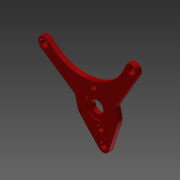
# Autodesk Inventor part: Part2
Saved by Autodesk Inventor 2014 SP1 (Build 180222100, 222)
## iProperties
Created: 2014-01-05
Part Number: Part2
Material: Aluminum 6061
Document SubType Name: Modeling
Designer: Rauhul Varma
Density: 2.71 g/cm^3
Appearance: Red
Mass: 9.68241 g
Surface Area: 32.817 cm^2
Volume: 3.57285 cm^3
Author: Rauhul Varma
Autodesk Inventor part; units mm, degrees
ref_plane "YZ Plane" through (0, 0, 0) normal (1, 0, 0) x (0, 1, 0)
ref_plane "XZ Plane" through (0, 0, 0) normal (0, 1, 0) x (-1, 0, 0)
ref_plane "XY Plane" through (0, 0, 0) normal (0, 0, 1) x (1, 0, 0)
sketch "Main Outline" plane through (0, 0, 0) normal (0, 0, 1) x (1, 0, 0)
  line L0 (0, 0) -> (304.8, 0) construction
  line L1 (304.8, 0) -> (304.8, 50.8) construction
  line L2 (304.8, 50.8) -> (0, 50.8) construction
  line L3 (0, 50.8) -> (0, 0) construction
  line L4 (0, 50.8) -> (0, 53.34) construction
  line L5 (0, 53.34) -> (304.8, 53.34) construction
  line L6 (304.8, 53.34) -> (304.8, 50.8) construction
  circle A0 centre (152.4, 23.8125) radius 17.4625 construction
  line L7 (152.4, 23.8125) -> (152.4, 0) construction
  circle A1 centre (152.4, 23.8125) radius 27.94 construction
  circle A2 centre (152.4, 23.8125) radius 21.59 construction
  line L8 (152.4, 23.8125) -> (144.1569, 60.2292) construction
  circle A3 centre (144.1569, 60.2292) radius 15.24 construction
  circle A4 centre (144.1569, 60.2292) radius 8.89 construction
  circle A5 centre (144.1569, 60.2292) radius 14.2875 construction
  arc A6 (163.8162, 72.0089) -> (128.198, 43.7805) centre (144.1569, 60.2292) ccw construction
  circle A7 centre (98.8106, 85.598) radius 32.258 construction
  circle A8 centre (124.5097, 147.0273) radius 32.258 construction
  circle A9 centre (174.158, 102.6533) radius 32.258 construction
  circle A10 centre (144.1569, 60.2292) radius 11.1125 construction
  circle A11 centre (152.4, 23.8125) radius 49.53 construction
  line L9 (144.1569, 60.2292) -> (124.5097, 147.0273) construction
  line L10 (144.1569, 60.2292) -> (98.8106, 85.598) construction
  line L11 (98.8106, 85.598) -> (174.158, 102.6533) construction
  line L12 (174.158, 102.6533) -> (144.1569, 60.2292) construction
  circle A12 centre (98.8106, 85.598) radius 9.5493 construction
  arc A13 (172.0498, 111.9669) -> (183.1109, 99.3313) centre (174.158, 102.6533) ccw construction
  circle A14 centre (124.5097, 147.0273) radius 9.5493 construction
  line L13 (96.7024, 94.9117) -> (172.0498, 111.9669) construction
  line L14 (183.1109, 99.3313) -> (165.6438, 52.2565) construction
  line L15 (92.161, 78.7444) -> (128.198, 43.7805) construction
  line L16 (172.0498, 111.9669) -> (174.158, 102.6533) construction
  line L17 (174.158, 102.6533) -> (183.1109, 99.3313) construction
  arc A15 (183.1109, 99.3313) -> (172.0498, 111.9669) centre (174.158, 102.6533) ccw construction
  arc A16 (165.6438, 52.2565) -> (163.8162, 72.0089) centre (144.1569, 60.2292) ccw construction
  arc A17 (128.198, 43.7805) -> (165.6438, 52.2565) centre (144.1569, 60.2292) ccw construction
  circle A18 centre (124.4396, 147.337) radius 32.258 construction
  circle A19 centre (124.3695, 147.6466) radius 32.258 construction
  circle A20 centre (124.2994, 147.9563) radius 32.258 construction
  line L18 (124.5097, 147.0273) -> (124.2994, 147.9563) construction
  circle A21 centre (124.5798, 146.7176) radius 32.258 construction
  circle A22 centre (117.4622, 43.2997) radius 9.525 construction
  circle A23 centre (175.54, 56.4459) radius 9.525 construction
  line L19 (152.4, 23.8125) -> (117.4622, 43.2997) construction
  line L20 (152.4, 23.8125) -> (175.54, 56.4459) construction
  line L21 (117.4622, 43.2997) -> (98.8106, 85.598) construction
  line L22 (175.54, 56.4459) -> (174.158, 102.6533) construction
  circle A24 centre (133.7342, 106.2753) radius 7.9375 construction
  line L23 (133.401, 150.5107) -> (165.496, 68.5894) construction
  circle A25 centre (152.4, 23.8125) radius 29.845 construction
  line L24 (114.985, 146.3422) -> (121.2977, 58.5849) construction
  circle A26 centre (99.0876, 85.443) radius 32.258 construction
  circle A27 centre (97.9793, 86.063) radius 32.258 construction
  line L25 (97.9793, 86.063) -> (98.8106, 85.598) construction
  circle A28 centre (98.2564, 85.908) radius 32.258 construction
  circle A29 centre (98.5335, 85.753) radius 32.258 construction
  circle A30 centre (152.4, 23.8125) radius 29.845 construction
  circle A31 centre (122.555, 23.8125) radius 6.35 construction
  circle A32 centre (179.3358, 36.6651) radius 6.35 construction
  line L26 (122.555, 23.8125) -> (152.4, 23.8125) construction
  line L27 (152.4, 23.8125) -> (182.245, 23.8125) construction
  circle A33 centre (182.245, 23.8125) radius 6.35 construction
  circle A34 centre (125.4642, 10.9599) radius 6.35 construction
  circle A35 centre (150.1885, 33.5827) radius 39.8623 construction
  line L28 (72.8944, 65.7819) -> (119.1902, 8.5205) construction
  circle A36 centre (174.708, 103.431) radius 32.258 construction
  line L29 (174.158, 102.6533) -> (174.708, 103.431) construction
  circle A37 centre (174.5246, 103.1717) radius 32.258 construction
  circle A38 centre (174.3413, 102.9125) radius 32.258 construction
  circle A39 centre (173.9747, 102.394) radius 32.258 construction
  line L30 (188.958, 24.3128) -> (206.0816, 95.9295) construction
  circle A40 centre (133.7342, 106.2753) radius 8.1693 construction
  arc A41 (85.4541, 115.7901) -> (94.2274, 135.7949) centre (79.2901, 130.4196) ccw construction
  arc A42 (156.6774, 149.9308) -> (173.2104, 135.6542) centre (172.4734, 151.5121) ccw construction
  line L31 (124.2994, 147.9563) -> (124.8602, 145.479) construction
  line L32 (114.3901, 145.7133) -> (114.9509, 143.236) construction
  line L33 (134.7695, 147.722) -> (134.2088, 150.1993) construction
  arc A43 (134.2088, 150.1993) -> (114.3901, 145.7133) centre (124.2994, 147.9563) ccw construction
  arc A44 (114.9509, 143.236) -> (134.7695, 147.722) centre (124.8602, 145.479) ccw construction
  line L34 (174.708, 103.431) -> (173.2414, 101.3571) construction
  line L35 (166.4126, 109.2972) -> (164.9461, 107.2234) construction
  line L36 (181.5368, 95.4909) -> (183.0033, 97.5647) construction
  arc A45 (183.0033, 97.5647) -> (166.4126, 109.2972) centre (174.708, 103.431) ccw construction
  arc A46 (164.9461, 107.2234) -> (181.5368, 95.4909) centre (173.2414, 101.3571) ccw construction
  line L37 (97.9793, 86.063) -> (100.196, 84.8229) construction
  line L38 (93.0188, 77.1963) -> (95.2355, 75.9562) construction
  line L39 (105.1564, 93.6897) -> (102.9398, 94.9298) construction
  arc A47 (102.9398, 94.9298) -> (93.0188, 77.1963) centre (97.9793, 86.063) ccw construction
  arc A48 (95.2355, 75.9562) -> (105.1564, 93.6897) centre (100.196, 84.8229) ccw construction
  circle A49 centre (117.4622, 43.2997) radius 3.9687 construction
  circle A50 centre (175.54, 56.4459) radius 3.9687 construction
  line L40 (152.4, 23.8125) -> (158.9889, -5.2961) construction
  arc A51 (89.3511, 54.6895) -> (85.9237, 49.6664) centre (88.3927, 51.6626) ccw construction
  arc A52 (201.2624, 75.7739) -> (196.006, 78.8314) centre (198.1744, 76.5122) ccw construction
  circle A53 centre (152.4, 23.8125) radius 14.224 construction
  circle A54 centre (133.7342, 106.2753) radius 3.9687 construction
  circle A55 centre (156.886, 3.9939) radius 6.35 construction
  circle A56 centre (156.886, 3.9939) radius 2.0828 construction
  circle A57 centre (152.4, 23.8125) radius 20.32 construction
  line L41 (132.9935, 29.8368) -> (152.4, 23.8125) construction
  line L42 (152.4, 23.8125) -> (167.3204, 37.6068) construction
  circle A58 centre (167.3204, 37.6068) radius 2.0828 construction
  circle A59 centre (167.3204, 37.6068) radius 3.9687 construction
  circle A60 centre (132.9935, 29.8368) radius 2.0828 construction
  circle A61 centre (132.9935, 29.8368) radius 3.9688 construction
  point P0 (173.9747, 102.394)
  point P1 (99.0876, 85.443)
  dimension "d18" = 99.06
  dimension "d58" = 64.516
  dimension "d86" = 64.516
  dimension "d0" = 304.8
  dimension "d1" = 50.8
  dimension "d2" = 2.54
  dimension "d3" = 34.925
  dimension "d4" = 23.8125
  dimension "d5" = 152.4
  dimension "d6" = 55.88
  dimension "d7" = 43.18
  dimension "d8" = 37.338
  dimension "d10" = 30.48
  dimension "d11" = 17.78
  dimension "d12" = 28.575
  dimension "d13" = 45.8366
  dimension "d14" = 64.516
  dimension "d15" = 64.516
  dimension "d16" = 64.516
  dimension "d17" = 22.225
  dimension "d19" = 51.9602
  dimension "d20" = 88.9939
  dimension "d21" = 19.0986
  dimension "d22" = 19.0986
  dimension "d23" = 19.0986
  dimension "d30" = 123.112
  dimension "d40" = 64.516
  dimension "d41" = 64.516
  dimension "d42" = 64.516
  dimension "d43" = 0.9525
  dimension "d44" = 0.3175
  dimension "d45" = 0.635
  dimension "d46" = 64.516
  dimension "d47" = 0.3175
  dimension "d48" = 19.05
  dimension "d49" = 19.05
  dimension "d50" = 40.005
  dimension "d51" = 40.005
  dimension "d52" = 46.228
  dimension "d54" = 46.228
  dimension "d55" = 15.875
  dimension "d56" = 41.4655
  dimension "d57" = 59.69
  dimension "d59" = 64.516
  dimension "d60" = 64.516
  dimension "d61" = 64.516
  dimension "d62" = 0.3175
  dimension "d63" = 0.3175
  dimension "d64" = 0.635
  dimension "d65" = 0.9525
  dimension "d73" = 12.7
  dimension "d74" = 12.7
  dimension "d76" = 59.69
  dimension "d78" = 12.7
  dimension "d79" = 12.7
  dimension "d80" = 64.516
  dimension "d81" = 0.9525
  dimension "d82" = 64.516
  dimension "d83" = 64.516
  dimension "d84" = 0.3175
  dimension "d85" = 0.635
  dimension "d88" = 0.3175
  dimension "d89" = 31.75
  dimension "d90" = 31.75
  dimension "d94" = 1.5875
  dimension "d95" = 20.32
  dimension "d96" = 1.5875
  constraints: 92 end point, 59 centre point, 54 point on circle, 38 tangent, 26 coincident, 16 point on line, 9 collinear, 6 parallel, 4 midpoint, 4 perpendicular, 3 symmetric about line, 2 horizontal, 13 other
  measures "d0" distance of L2.end L1.end
  measures "d1" distance of L1.end L0.end
  measures "d2" distance of L2.end L4.end
  measures "d3" diameter of A0
  measures "d4" distance of L7.start L7.end
  measures "d5" distance between parallel lines of L3 L7
  measures "d6" diameter of A1
  measures "d7" diameter of A2
  measures "d8" distance of L8.start L8.end
  measures "d10" diameter of A3
  measures "d11" diameter of A4
  measures "d12" diameter of A5
  measures "d13" diameter of A6
  measures "d14" diameter of A7
  measures "d15" diameter of A8
  measures "d16" diameter of A9
  measures "d17" diameter of A10
  measures "d19" distance of L9.start L10.end
  measures "d20" distance of L9.start L9.end
  measures "d21" diameter of A12
  measures "d22" diameter of A13
  measures "d23" diameter of A14
  measures "d30" angle of L17 L16
  measures "d40" diameter of A18
  measures "d41" diameter of A19
  measures "d42" diameter of A20
  measures "d43" distance of L18.end L9.end
  measures "d44" distance of A18.centre L9.end
  measures "d45" distance of A19.centre L9.end
  measures "d46" diameter of A21
  measures "d47" distance of L9.end A21.centre
  measures "d48" diameter of A22
  measures "d49" diameter of A23
  measures "d50" distance of L19.start L19.end
  measures "d51" distance of L19.start L20.end
  measures "d52" distance of L19.end L21.end
  measures "d54" distance of L20.end L16.end
  measures "d55" diameter of A24
  measures "d56" distance of A21.centre A24.centre
  measures "d57" diameter of A25
  measures "d59" diameter of A27
  measures "d60" diameter of A28
  measures "d61" diameter of A29
  measures "d62" distance of point (99.088, 85.443) L10.end
  measures "d63" distance of L10.end A29.centre
  measures "d64" distance of L10.end A28.centre
  measures "d65" distance of L25.start L10.end
  measures "d73" diameter of A31
  measures "d74" diameter of A32
  measures "d76" diameter of A30
  measures "d78" diameter of A33
  measures "d79" diameter of A34
  measures "d80" diameter of A36
  measures "d81" distance of L29.start L29.end
  measures "d82" diameter of A37
  measures "d83" diameter of A38
  measures "d84" distance of L16.end A38.centre
  measures "d85" distance of L11.end A37.centre
  measures "d88" distance of L11.end point (173.975, 102.394)
  measures "d89" diameter of A41
  measures "d90" diameter of A42
  measures "d94" distance of L9.end L31.end
  measures "d95" diameter of A44
  measures "d96" distance of L11.end L34.end
sketch "Upper CIM C-C Check" plane through (0, 0, 0) normal (0, 0, 1) x (1, 0, 0)
  arc A0 (3.4429, -22.6582) -> (3.4429, 22.6582) centre (0, 0) ccw construction
  arc A1 (90.4285, 9.4409) -> (90.4285, -9.4409) centre (88.9939, 0) ccw construction
  line L0 (88.9939, 0) -> (0, 0) construction
  line L1 (90.4285, 9.4409) -> (3.4429, 22.6582)
  line L2 (3.4429, -22.6582) -> (90.4285, -9.4409)
  arc A2 (90.4285, -9.4409) -> (90.4285, 9.4409) centre (88.9939, 0) ccw
  arc A3 (3.4429, 22.6582) -> (3.4429, -22.6582) centre (0, 0) ccw
  dimension "d24" = 45.8366
  dimension "d25" = 19.0986
  dimension "d26" = 78.9119
  dimension "d27" = 87.984
  dimension "d28" = 27.12
  dimension "d29" = 88.9939
  constraints: 8 point on circle, 6 end point, 4 centre point, 4 tangent, 1 coincident, 1 horizontal
  measures "d24" diameter of A0
  measures "d25" diameter of A1
  measures "d27" distance of L1.start L1.end
  measures "d29" distance of L0.start L0.end
sketch "Sketch3" plane through (0, 0, 0) normal (0, 0, 1) x (1, 0, 0)
  arc A0 (120.2749, 46.0997) -> (115.2358, 40.0143) centre (117.4622, 43.2997) ccw
  arc A1 (178.9642, 54.4395) -> (171.7957, 57.7617) centre (175.54, 56.4459) ccw
  arc A2 (160.6699, 2.7967) -> (153.9865, 1.2839) centre (156.886, 3.9939) ccw construction
  arc A3 (128.198, 43.7805) -> (165.6438, 52.2565) centre (144.1569, 60.2292) ccw construction
  arc A4 (139.8542, 17.11) -> (142.0082, 14.1) centre (152.4, 23.8125) ccw
  line L0 (156.886, 3.9939) -> (144.1569, 60.2292) construction
  circle A5 centre (152.4, 23.8125) radius 11.176 construction
  line L1 (166.6093, 23.1661) -> (164.9458, 30.515)
  line L2 (160.6699, 2.7967) -> (165.9615, 19.5219)
  line L3 (164.9458, 30.515) -> (178.9642, 54.4395)
  line L4 (138.1907, 24.4589) -> (139.8542, 17.11)
  line L5 (142.0082, 14.1) -> (153.9865, 1.2839)
  line L6 (138.1907, 24.4589) -> (115.2358, 40.0143)
  arc A6 (138.1907, 24.4589) -> (139.8542, 17.11) centre (152.4, 23.8125) ccw construction
  arc A7 (164.9458, 30.515) -> (138.1907, 24.4589) centre (152.4, 23.8125) ccw construction
  arc A8 (166.6093, 23.1661) -> (164.9458, 30.515) centre (152.4, 23.8125) ccw construction
  arc A9 (155.5402, 9.9395) -> (165.9615, 19.5219) centre (152.4, 23.8125) ccw construction
  arc A10 (142.0082, 14.1) -> (155.5402, 9.9395) centre (152.4, 23.8125) ccw construction
  arc A11 (165.9615, 19.5219) -> (166.6093, 23.1661) centre (152.4, 23.8125) ccw
  arc A12 (153.9865, 1.2839) -> (160.6699, 2.7967) centre (156.886, 3.9939) ccw
  arc A13 (120.2749, 46.0997) -> (171.7957, 57.7617) centre (142.3753, 68.1002) ccw
  arc A14 (171.7957, 57.7617) -> (120.2749, 46.0997) centre (142.3753, 68.1002) ccw construction
  arc A15 (115.2358, 40.0143) -> (120.2749, 46.0997) centre (117.4622, 43.2997) ccw construction
  arc A16 (171.7957, 57.7617) -> (178.9642, 54.4395) centre (175.54, 56.4459) ccw construction
  circle A17 centre (152.4, 23.8125) radius 3.9688
  point P0 (0, 0)
  point P1 (149.9327, 34.7127)
  point P2 (154.8673, 12.9123)
  dimension "d115" = 7.9375
  dimension "d117" = 22.352
  dimension "d118" = 13.716
  dimension "d119" = 13.716
  dimension "d120" = 14.224
  dimension "d121" = 7.9375
  constraints: 39 point on circle, 17 centre point, 17 tangent, 14 end point, 7 coincident, 3 point on line, 2 equal radius, 2 parallel
  measures "d115" diameter of A0
  measures "d117" diameter of A5
  measures "d118" distance from line of point (152.4, 23.812) L1
  measures "d119" distance from line of point (152.4, 23.812) L4
  measures "d120" radius of A7
  measures "d121" diameter of A17
extrude "Extrusion1" add sketch "Sketch3" along normal blind 3.175
hole "Hole1" at (175.54, 56.4459, 0) at (117.4622, 43.2997, 0) direction (0, 0, 1) diameter 4.9784 end through all clearance for "Socket Head Cap Screw" size "#10" standard "Ansi Unified Screw Threads"
hole "Hole2" at (149.9327, 34.7127, 0) at (154.8673, 12.9123, 0) direction (0, 0, 1) diameter 4.2164 end through all
hole "Hole3" at (156.886, 3.9939, 0) direction (0, 0, 1) diameter 4.318 end through all clearance for "Socket Head Cap Screw" size "#8" standard "Ansi Unified Screw Threads"
fillet "Fillet1" radius 3.175 4 edges at (138.1907, 24.4589, 1.5875) (164.9458, 30.515, 1.5875) (166.6093, 23.1661, 1.5875) (139.8542, 17.11, 1.5875)
sketch "Sketch4" plane through (0, 0, 3.175) normal (0, 0, 1) x (1, 0, 0)
  circle A0 centre (152.4, 23.8125) radius 3.9687 projected
  arc A1 (165.9615, 19.5219) -> (166.5764, 22.6501) centre (152.4, 23.8125) ccw projected
  circle A2 centre (152.4, 23.8125) radius 7.1437
  point P0 (0, 0)
  dimension "d146" = 14.2875
  constraints: 1 centre point, 1 coincident
  measures "d146" diameter of A2
extrude "Extrusion2" cut sketch "Sketch4" against normal blind 0.635
equation "\"d3\" = r10"
equation "\"d6\" = g44"
equation "\"d7\" = g34"
equation "\"d10\" = g24"
equation "\"d11\" = g14"
equation "\"d12\" = r8"
equation "\"d13\" = p48"
equation "\"d14\" = cim"
equation "\"d15\" = cim"
equation "\"d16\" = cim"
equation "\"d17\" = r6"
equation "\"d21\" = p20"
equation "\"d22\" = p20"
equation "\"d23\" = p20"
equation "\"d24\" = p48"
equation "\"d25\" = p20"
equation "\"d29\" = d20"
equation "\"g14\" = 17.78"
equation "\"g24\" = 30.48"
equation "\"g34\" = 43.18"
equation "\"g44\" = 55.88"
equation "\"p20\" = 19.09859"
equation "\"p48\" = 45.83662"
equation "\"r10\" = 34.925"
equation "\"r9\" = 31.75"
equation "\"r8\" = 28.575"
equation "\"r7\" = 25.4"
equation "\"r6\" = 22.225"
equation "\"r5\" = 19.05"
equation "\"r4\" = 15.875"
equation "\"r3\" = 12.7"
equation "\"cim\" = 64.516"
equation "\"act\" = 28.448"
equation "\"actL\" = 23.749"
equation "\"UpperCimCCCheck\" = 2 * d27 + d26 + d28"
equation "\"LowerBeltPathCCCheck\" = 267"
body "Solid1"
